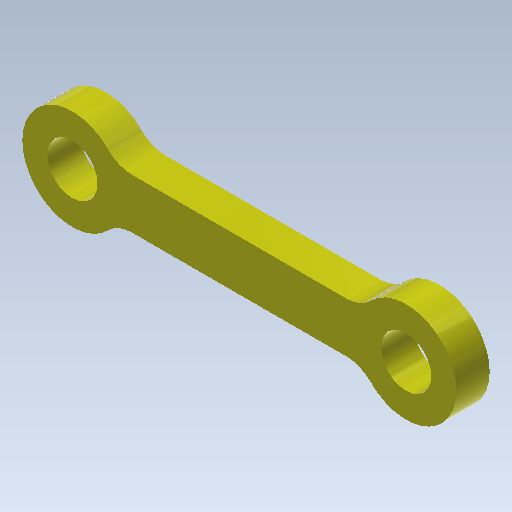
# Autodesk Inventor part: Bar1
Saved by Autodesk Inventor 2021 (Build 250183000, 183)
## iProperties
Created: 2010-08-06
Part Number: Bar1
Document SubType Name: Modeling
Designer: nguyenducthang
Density: 1 g/cm^3
Mass: 0.0214154 g
Surface Area: 0.824931 cm^2
Volume: 0.0214154 cm^3
Material: Generic
Appearance: Smooth - Yellow
Author: nguyenducthang
Autodesk Inventor part; units mm, degrees
ref_plane "YZ Plane" through (0, 0, 0) normal (1, 0, 0) x (0, 1, 0)
ref_plane "XZ Plane" through (0, 0, 0) normal (0, 1, 0) x (-1, 0, 0)
ref_plane "XY Plane" through (0, 0, 0) normal (0, 0, 1) x (1, 0, 0)
sketch "Sketch3" plane through (0, 0, 0) normal (0, 0, 1) x (1, 0, 0)
  circle A0 centre (0, 0) radius 0.75
  line L0 (0, 0) -> (80, 0) construction
  circle A1 centre (10, 0) radius 0.75
  circle A2 centre (0, 0) radius 1.5
  circle A3 centre (10, 0) radius 1.5
  line L1 (1.299, 0.75) -> (8.701, 0.75)
  line L2 (1.299, -0.75) -> (8.701, -0.75)
  dimension "d10" = 1.5
  dimension "d20" = 10
  dimension "d21" = 3
  dimension "d26" = 0.75
  constraints: 6 end point, 4 centre point, 4 point on circle, 3 coincident, 2 equal radius, 1 horizontal, 1 parallel, 1 point on line, 2 other
  measures "d10" diameter of A0
  measures "d20" distance of A0.centre A1.centre
  measures "d21" diameter of A2
  measures "d26" distance between parallel lines of L1 L0
extrude "Extrusion3" add sketch "Sketch3" along normal blind 1
fillet "Fillet1" radius 1 4 edges at (1.299, 0.75, 0.5) (1.299, -0.75, 0.5) (8.701, 0.75, 0.5) (8.701, -0.75, 0.5)
body "Solid1"
